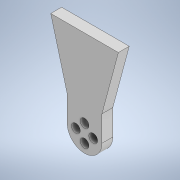
# Autodesk Inventor part: OutPut_Shaft_From_Gearbox
Saved by Autodesk Inventor 2022 (Build 260153000, 153)
## iProperties
Created: 2022-01-20
Part Number: OutPut_Shaft_From_Gearbox
Material: Generic
Document SubType Name: Modeling
Designer: Mlees
Density: 1 g/cm^3
Appearance: Default
Author: Mlees
Autodesk Inventor part; units mm, degrees
ref_plane "YZ Plane" through (0, 0, 0) normal (1, 0, 0) x (0, 1, 0)
ref_plane "XZ Plane" through (0, 0, 0) normal (0, 1, 0) x (-1, 0, 0)
ref_plane "XY Plane" through (0, 0, 0) normal (0, 0, 1) x (1, 0, 0)
sketch "Sketch1" plane through (0, 0, 0) normal (0, 0, 1) x (1, 0, 0)
  circle A0 centre (0, 4) radius 2
  circle A1 centre (-4, 0) radius 2
  circle A2 centre (0, -4) radius 2
  circle A3 centre (4, 0) radius 2
  line L0 (7, 40) -> (-7, 40)
  line L1 (8, 11.7321) -> (15.5744, 40)
  line L2 (7, 8) -> (40.1288, 8) construction
  line L3 (15.5744, 40) -> (7, 40)
  line L4 (-8, 11.7321) -> (-15.5744, 40)
  line L5 (-15.5744, 40) -> (-7, 40)
  line L6 (8, 0) -> (8, 11.7321)
  line L7 (-8, 0) -> (-8, 11.7321)
  arc A4 (-8, 0) -> (8, 0) centre (0, 0) ccw
  dimension "d2" = 4
  dimension "d5" = 360
  constraints: 16 end point, 5 centre point, 2 point on circle, 1 horizontal, 9 other
  measures "d2" diameter of A0
extrude "Extrusion1" add sketch "Sketch1" along normal blind 5
sketch "Sketch2" plane through (0, 0, 0) normal (0, 0, -1) x (-1, 0, 0)
  circle A0 centre (0, 0) radius 6.625
  dimension "d18" = 13.25
  constraints: 1 centre point, 1 coincident
  measures "d18" diameter of A0
extrude "Extrusion2" cut sketch "Sketch2" against normal blind 2
body "Solid1"
